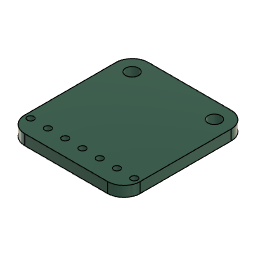
BME280 v2 (Autodesk Fusion 360 design; units mm, degrees)
Autodesk Fusion 360 part; units mm, degrees
sketch "Skizze1" plane through (0, 0, 0) normal (0, 0, 1) x (1, 0, 0)
  line L0 (2.5, 0) -> (15.28, 0)
  line L1 (17.78, 2.5) -> (17.78, 16.55)
  line L2 (15.28, 19.05) -> (2.5, 19.05)
  line L3 (0, 16.55) -> (0, 2.5)
  arc A0 (2.5, 19.05) -> (0, 16.55) centre (2.5, 16.55) ccw
  arc A1 (17.78, 16.55) -> (15.28, 19.05) centre (15.28, 16.55) ccw
  arc A2 (15.28, 0) -> (17.78, 2.5) centre (15.28, 2.5) ccw
  arc A3 (0, 2.5) -> (2.5, 0) centre (2.5, 2.5) ccw
  circle A4 centre (2.5, 16.55) radius 1
  circle A5 centre (15.2, 16.55) radius 1
  circle A6 centre (0.89, 2.5) radius 0.5
  circle A7 centre (3.5567, 2.5) radius 0.5
  circle A8 centre (6.2233, 2.5) radius 0.5
  circle A9 centre (8.89, 2.5) radius 0.5
  circle A10 centre (11.5567, 2.5) radius 0.5
  circle A11 centre (14.2233, 2.5) radius 0.5
  circle A12 centre (16.89, 2.5) radius 0.5
  point P0 (17.78, 0)
  dimension "d3" = 17.78
  dimension "d4" = 19.05
  dimension "d5" = 2.5
  dimension "d6" = 2
  dimension "d9" = 12.7
  dimension "d10" = 0
  dimension "d11" = 1
  dimension "d12" = 2.5
  dimension "d15" = 16
  dimension "d16" = 0
  dimension "d17" = 8.89
  constraint horizontal L0
  constraint vertical L1
  constraint horizontal L2
  constraint vertical L3
  constraint tangent L2 A0
  constraint tangent L3 A0
  constraint tangent L1 A1
  constraint tangent L2 A1
  constraint equal A0 A1
  constraint coincident P0 L0
  constraint coincident P0 L1
  constraint tangent L0 A2
  constraint tangent L1 A2
  constraint equal A0 A2
  constraint coincident origin L0
  constraint coincident origin L3
  constraint tangent L0 A3
  constraint tangent L3 A3
  constraint equal A0 A3
  constraint concentric A0 A4
  measures "d3" distance of origin P0
  measures "d4" distance of L0 L2
  measures "d5" radius of A0
  measures "d6" diameter of A4
  measures "d11" diameter of A6
  measures "d12" distance of L0 A6.centre
  measures "d17" distance of L3 A9.centre
extrude "Extrusion1" add sketch "Skizze1" along normal blind 1.6
